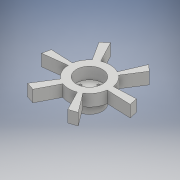
# Autodesk Inventor part: carroussel
Saved by Autodesk Inventor 2017 (Build 210142000, 142)
## iProperties
Part Number: carroussel
Material: Générique
Document SubType Name: Modeling
Designer: Thomas
Density: 1 g/cm^3
Appearance: Par défaut
Author: Thomas
Autodesk Inventor part; units mm, degrees
ref_plane "YZ Plane" through (0, 0, 0) normal (1, 0, 0) x (0, 1, 0)
ref_plane "XZ Plane" through (0, 0, 0) normal (0, 1, 0) x (-1, 0, 0)
ref_plane "XY Plane" through (0, 0, 0) normal (0, 0, 1) x (1, 0, 0)
sketch "Esquisse1" plane through (0, 0, 0) normal (0, 0, 1) x (1, 0, 0)
  circle A0 centre (0, 0) radius 1.35
  circle A1 centre (0, -7.75) radius 1.15
  circle A2 centre (7.75, 0) radius 1.15
  circle A3 centre (0, 7.75) radius 1.15
  circle A4 centre (-7.75, 0) radius 1.15
  circle A5 centre (0, 0) radius 11
  constraints: 6 centre point
extrude "Extrusion1" add sketch "Esquisse1" along normal blind 10
sketch "Esquisse2" plane through (0, 0, 10) normal (0, 0, 1) x (1, 0, 0)
  circle A0 centre (0, 0) radius 1.35 projected
  circle A1 centre (-7.75, 0) radius 1.15 projected
  circle A2 centre (0, 7.75) radius 1.15 projected
  circle A3 centre (7.75, 0) radius 1.15 projected
  circle A4 centre (0, -7.75) radius 1.15 projected
  circle A5 centre (0, 0) radius 11 projected
  circle A6 centre (-50.0425, 0) radius 22.5 construction
  circle A7 centre (0, -50.0425) radius 22.5 construction
  circle A8 centre (50.0425, 0) radius 22.5 construction
  circle A9 centre (0, 50.0425) radius 22.5 construction
  circle A10 centre (0, 0) radius 1.35 projected
  line L0 (0, 50.0425) -> (-56.3346, 50.0425) construction
  line L1 (-56.3346, 50.0425) -> (72.5425, 50.0425) construction
  circle A11 centre (45, 50.0425) radius 22.5 construction
  circle A12 centre (90, 50.0425) radius 22.5 construction
  circle A13 centre (-45, 50.0425) radius 22.5 construction
  circle A14 centre (-90, 50.0425) radius 22.5 construction
  circle A15 centre (0, 0) radius 11 projected
  line L2 (-16.2007, 34.167) -> (-21.379, 29.4772)
  line L3 (0, 0) -> (0, 23.6812) construction
  line L4 (8.1922, 15.4641) -> (16.2007, 34.167)
  line L5 (16.2007, 34.167) -> (21.379, 29.4772)
  line L6 (21.379, 29.4772) -> (11.2487, 13.5828)
  line L7 (-6.6711, 16.1786) -> (-16.2007, 34.167)
  line L8 (-21.379, 29.4772) -> (-11.2487, 13.5828)
  line L9 (-21.4892, -31.1137) -> (-14.8385, -33.2533)
  line L10 (-10.6755, -13.8667) -> (-21.4892, -31.1137)
  line L11 (-14.8385, -33.2533) -> (-6.1388, -16.533)
  line L12 (-17.4884, -0.6374) -> (-37.6898, -3.0533)
  line L13 (-36.2175, 3.7762) -> (-17.3874, 2.9502)
  line L14 (-37.6898, -3.0533) -> (-36.2175, 3.7762)
  line L15 (37.6898, -3.0533) -> (36.2175, 3.7762)
  line L16 (17.3466, -2.3119) -> (37.6898, -3.0533)
  line L17 (36.2175, 3.7762) -> (17.3874, 2.9502)
  line L18 (9.2962, -14.8267) -> (21.4892, -31.1137)
  line L19 (14.8385, -33.2533) -> (6.1388, -16.533)
  line L20 (21.4892, -31.1137) -> (14.8385, -33.2533)
  arc A16 (8.1922, 15.4641) -> (-6.6711, 16.1786) centre (0, 0) ccw
  arc A17 (17.3874, 2.9502) -> (11.2487, 13.5828) centre (0, 0) ccw
  arc A18 (9.2962, -14.8267) -> (17.3466, -2.3119) centre (0, 0) ccw
  arc A19 (-6.1388, -16.533) -> (6.1388, -16.533) centre (0, 0) ccw
  arc A20 (-11.2487, 13.5828) -> (-17.3874, 2.9502) centre (0, 0) ccw
  arc A21 (-17.4884, -0.6374) -> (-10.6755, -13.8667) centre (0, 0) ccw
  dimension "d2" = 45
  dimension "d5" = 360
  dimension "d10" = 45
  dimension "d17" = 45
  dimension "d24" = 240
  constraints: 42 end point, 14 centre point, 12 point on circle, 3 horizontal, 2 symmetric about line, 1 coincident, 1 point on line, 1 vertical, 46 other
  measures "d2" diameter of A6
  measures "d10" distance of L0.start A11.centre
  measures "d17" distance of L0.start A13.centre
extrude "Extrusion2" add sketch "Esquisse2" along normal blind 10 contours L7 A16 L4 L5 L6 A17 L17 L15 L16 A18 L18 L20 L19 A19 L11 L9 L10 A21 L12 L14 L13 A20 L8 L2
